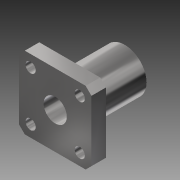
# Autodesk Inventor part: lm8kuu
Saved by Autodesk Inventor 2014 (Build 180170000, 170)
## iProperties
Created: 2014-07-14
Part Number: lm8kuu
Material: Generic
Document SubType Name: Modeling
Designer: cruiser
Density: 1 g/cm^3
Appearance: Stainless - Polished
Author: cruiser
Autodesk Inventor part; units mm, degrees
ref_plane "YZ Plane" through (0, 0, 0) normal (1, 0, 0) x (0, 1, 0)
ref_plane "XZ Plane" through (0, 0, 0) normal (0, 1, 0) x (-1, 0, 0)
ref_plane "XY Plane" through (0, 0, 0) normal (0, 0, 1) x (1, 0, 0)
sketch "Sketch1" plane through (0, 0, 0) normal (0, 1, 0) x (-1, 0, 0)
  line L0 (10, -12) -> (-10, -12)
  line L1 (-12, -10) -> (-12, 10)
  line L2 (-10, 12) -> (10, 12)
  line L3 (12, 10) -> (12, -10)
  line L4 (12, -12) -> (-12, 12) construction
  line L5 (-12, -12) -> (12, 12) construction
  line L6 (8.4853, -8.4853) -> (6.7353, -8.4853)
  line L7 (-8.4853, -8.4853) -> (-8.4853, -6.7353)
  line L8 (-8.4853, 8.4853) -> (-6.7353, 8.4853)
  line L9 (8.4853, 8.4853) -> (8.4853, 6.7353)
  line L10 (8.4853, -8.4853) -> (-8.4853, 8.4853) construction
  line L11 (-8.4853, -8.4853) -> (8.4853, 8.4853) construction
  circle A0 centre (-8.4853, 8.4853) radius 1.75
  circle A1 centre (8.4853, 8.4853) radius 1.75
  circle A2 centre (-8.4853, -8.4853) radius 1.75
  circle A3 centre (8.4853, -8.4853) radius 1.75
  line L12 (-10, 12) -> (-12, 10)
  line L13 (-12, -10) -> (-10, -12)
  line L14 (10, -12) -> (12, -10)
  line L15 (10, 12) -> (12, 10)
  line L16 (-6.7353, 8.4853) -> (6.7353, 8.4853)
  line L17 (6.7353, 8.4853) -> (8.4853, 8.4853)
  line L18 (-8.4853, 6.7353) -> (-8.4853, 8.4853)
  line L19 (-8.4853, -6.7353) -> (-8.4853, 6.7353)
  line L20 (-6.7353, -8.4853) -> (-8.4853, -8.4853)
  line L21 (6.7353, -8.4853) -> (-6.7353, -8.4853)
  line L22 (8.4853, -6.7353) -> (8.4853, -8.4853)
  line L23 (8.4853, 6.7353) -> (8.4853, -6.7353)
  point P0 (0, 0)
  dimension "d0" = 24
  dimension "d1" = 24
  dimension "d2" = 12
  dimension "d3" = 3.5
  dimension "d4" = 3.5
  dimension "d5" = 3.5
  dimension "d6" = 3.5
  dimension "d7" = 2
  dimension "d8" = 2
  dimension "d9" = 2
  dimension "d10" = 2
  dimension "d11" = 2
  dimension "d12" = 2
  dimension "d13" = 2
  dimension "d14" = 2
  constraints: 48 end point, 20 parallel, 10 perpendicular, 9 point on line, 8 point on circle, 4 centre point, 4 coincident, 4 horizontal, 4 midpoint
  measures "d0" distance of L4.end L5.end
  measures "d1" distance of L5.start L4.end
  measures "d2" distance of point (0, 0) L8.start
  measures "d3" diameter of A0
  measures "d4" diameter of A1
  measures "d5" diameter of A2
  measures "d6" diameter of A3
  measures "d7" distance of L2.start L4.end
  measures "d8" distance of L1.end L4.end
  measures "d9" distance of L1.start L5.start
  measures "d10" distance of L0.end L5.start
  measures "d11" distance of L0.start L4.start
  measures "d12" distance of L3.end L4.start
  measures "d13" distance of L2.end L5.end
  measures "d14" distance of L3.start L5.end
extrude "Extrusion1" add sketch "Sketch1" along normal blind 5 contours L0 L13 L1 L12 L2 L15 L3 L14 | L21 A2 L19 A0 L16 A1 L23 A3
sketch "Sketch2" plane through (0, 5, 0) normal (0, 1, 0) x (1, 0, 0)
  circle A0 centre (0, 0) radius 6
  dimension "d17" = 12
  constraints: 1 centre point, 1 coincident
  measures "d17" diameter of A0
extrude "Extrusion2" add sketch "Sketch2" along normal blind 19
sketch "Sketch3" plane through (0, 24, 0) normal (0, 1, 0) x (1, 0, 0)
  circle A0 centre (0, 0) radius 6 projected
  circle A1 centre (0, 0) radius 4
  dimension "d20" = 8
  constraints: 1 centre point, 1 coincident
  measures "d20" diameter of A1
extrude "Extrusion3" cut sketch "Sketch3" against normal through all contours A1
equation "\"d8\" = d7"
equation "\"d9\" = d7"
equation "\"d10\" = d9"
equation "\"d11\" = d7"
equation "\"d12\" = d11"
equation "\"d13\" = d7"
equation "\"d14\" = d13"
body "Solid1"
